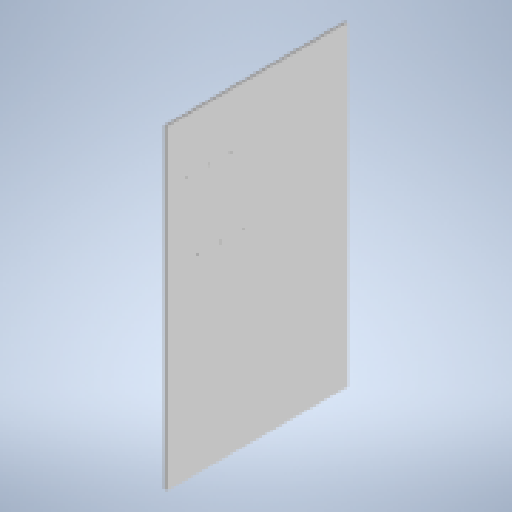
# Autodesk Inventor part: RT_ELE_MC_017_MainBackPlate
Saved by Autodesk Inventor 2025.4 (Build 294407000, 407)
## iProperties
Created: 2026-07-07
Part Number: RT_ELE_MC_017_MainBackPlate
Material: Générique
Document SubType Name: Modeling
Designer: louis
Density: 1 g/cm^3
Appearance: Par défaut
Author: louis
Autodesk Inventor part; units mm, degrees
ref_plane "YZ Plane" through (0, 0, 0) normal (1, 0, 0) x (0, 1, 0)
ref_plane "XZ Plane" through (0, 0, 0) normal (0, 1, 0) x (-1, 0, 0)
ref_plane "XY Plane" through (0, 0, 0) normal (0, 0, 1) x (1, 0, 0)
sketch "Sketch2" plane through (0, 0, 0) normal (1, 0, 0) x (0, 1, 0)
  line L0 (-200, 350) -> (200, 350)
  line L1 (200, 350) -> (200, -350)
  line L2 (200, -350) -> (-200, -350)
  line L3 (-200, -350) -> (-200, 350)
  line L4 (-200, 350) -> (200, -350) construction
  line L5 (200, 350) -> (-200, -350) construction
  point P0 (0, 0)
  dimension "d0" = 400
  dimension "d1" = 700
  constraints: 12 end point, 2 midpoint, 2 parallel, 1 horizontal, 1 perpendicular
  measures "d0" distance of L1.end L2.end
  measures "d1" distance of L0.end L1.end
extrude "Extrusion1" add sketch "Sketch2" along normal mid plane 6
sketch "Sketch3" plane through (3, 0, 0) normal (1, 0, 0) x (0, 0, -1)
  line L0 (350, -200) -> (350, 200) projected
  line L1 (350, 200) -> (-350, 200) projected
  line L2 (-350, 200) -> (-350, -200) projected
  line L3 (-350, -200) -> (350, -200) projected
  line L4 (-325, -175) -> (-325, 175)
  line L5 (-325, 175) -> (325, 175)
  line L6 (325, 175) -> (325, -175)
  line L7 (325, -175) -> (-325, -175)
  line L8 (-230.5, -159) -> (-230.5, -109) construction
  line L9 (-230.5, -109) -> (-230.5, -59) construction
  line L10 (-230.5, -159) -> (-69.5, -131) construction
  line L11 (-230.5, -109) -> (-69.5, -81) construction
  line L12 (-230.5, -59) -> (-69.5, -31) construction
  line L13 (-235, -165) -> (-65, -165)
  line L14 (-65, -165) -> (-65, -125)
  line L15 (-65, -125) -> (-235, -125)
  line L16 (-235, -125) -> (-235, -165)
  line L17 (-235, -165) -> (-65, -125) construction
  line L18 (-65, -165) -> (-235, -125) construction
  line L19 (-235, -115) -> (-65, -115)
  line L20 (-65, -115) -> (-65, -75)
  line L21 (-65, -75) -> (-235, -75)
  line L22 (-235, -75) -> (-235, -115)
  line L23 (-235, -115) -> (-65, -75) construction
  line L24 (-65, -115) -> (-235, -75) construction
  line L25 (-235, -65) -> (-65, -65)
  line L26 (-65, -65) -> (-65, -25)
  line L27 (-65, -25) -> (-235, -25)
  line L28 (-235, -25) -> (-235, -65)
  line L29 (-235, -65) -> (-65, -25) construction
  line L30 (-65, -65) -> (-235, -25) construction
  point P0 (0, 0)
  point P1 (-150, -145)
  point P2 (-150, -95)
  point P3 (-150, -45)
  dimension "d4" = 25
  dimension "d5" = 28
  dimension "d6" = 161
  dimension "d7" = 161
  dimension "d8" = 28
  dimension "d9" = 28
  dimension "d10" = 161
  dimension "d11" = 50
  dimension "d12" = 50
  dimension "d13" = 170
  dimension "d14" = 40
  dimension "d15" = 170
  dimension "d16" = 40
  dimension "d17" = 170
  dimension "d18" = 40
  dimension "d21" = 10
  dimension "d29" = 90
  constraints: 54 end point, 9 midpoint, 6 parallel, 3 horizontal, 3 perpendicular, 2 vertical, 3 other
  measures "d4" distance between parallel lines of L2 L4
  measures "d5" vertical distance of L10.end L8.start
  measures "d6" horizontal distance of L8.start L10.end
  measures "d7" horizontal distance of L11.end L9.start
  measures "d8" vertical distance of L11.end L9.start
  measures "d9" vertical distance of L12.end L12.start
  measures "d10" horizontal distance of L12.end L12.start
  measures "d11" distance of L8.start L9.start
  measures "d12" distance of L9.start L12.start
  measures "d13" distance of L15.end L14.end
  measures "d14" distance of L14.end L13.end
  measures "d15" distance of L21.end L21.start
  measures "d16" distance of L21.start L20.start
  measures "d17" distance of L27.end L27.start
  measures "d18" distance of L27.start L25.end
  measures "d21" distance between parallel lines of L7 L13
  measures "d29" horizontal distance of L4.start L13.start
hole "Hole1" at (3, -59, 230.5) at (3, -31, 69.5) at (3, -109, 230.5) at (3, -81, 69.5) at (3, -159, 230.5) at (3, -131, 69.5) direction (-1, 0, 0) diameter 4.5 end through all clearance for "Flat Head Machine Screw" size "M4" standard "Ansi Metric M Profile"
body "Solid1"
